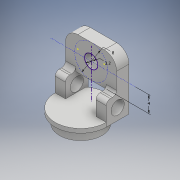
# Autodesk Inventor part: magnet-holder-end
Saved by Autodesk Inventor 2018 (Build 220112000, 112)
## iProperties
Created: 2025-03-13
Part Number: magnet-holder-end
Material: Generic
Document SubType Name: Modeling
Designer: neo
Density: 1 g/cm^3
Appearance: Default
Author: neo
Autodesk Inventor part; units mm, degrees
ref_plane "YZ Plane" through (0, 0, 0) normal (1, 0, 0) x (0, 1, 0)
ref_plane "XZ Plane" through (0, 0, 0) normal (0, 1, 0) x (-1, 0, 0)
ref_plane "XY Plane" through (0, 0, 0) normal (0, 0, 1) x (1, 0, 0)
sketch "Sketch1" plane through (0, 0, 0) normal (0, 0, 1) x (1, 0, 0)
  circle A0 centre (0, 0) radius 5.15
  dimension "d0" = 10.3
  constraints: 1 centre point, 1 coincident
  measures "d0" diameter of A0
extrude "Extrusion1" add sketch "Sketch1" along normal blind 2.3
sketch "Sketch2" plane through (0, 0, 2.3) normal (0, 0, 1) x (1, 0, 0)
  circle A0 centre (0, 0) radius 6.2
  dimension "d3" = 12.4
  constraints: 1 centre point, 1 coincident
  measures "d3" diameter of A0
extrude "Extrusion2" add sketch "Sketch2" along normal blind 1
sketch "Sketch3" plane through (0, 0, 2.3) normal (0, 0, -1) x (-1, 0, 0)
  circle A0 centre (0, 0) radius 6.2 construction
  line L0 (6.2, 0) -> (3.7, 0)
  line L1 (3.7, 0) -> (3.7, 5.5)
  line L2 (3.7, 5.5) -> (6.2, 5.5)
  line L3 (6.2, 5.5) -> (6.2, 0)
  line L4 (0, -6.2) -> (0, 6.2)
  circle A1 centre (0, 0) radius 6.2 construction
  line L5 (-6.2, 0) -> (-3.7, 0)
  line L6 (-3.7, 0) -> (-3.7, 5.5)
  line L7 (-3.7, 5.5) -> (-6.2, 5.5)
  line L8 (-6.2, 5.5) -> (-6.2, 0)
  dimension "d6" = 5.5
  dimension "d7" = 2.5
  constraints: 18 end point, 4 symmetric about line, 3 point on circle, 2 parallel, 1 horizontal, 1 horizontal alignment, 1 line through centre, 1 perpendicular, 1 vertical, 2 other
  measures "d6" distance of L2.end L0.start
  measures "d7" distance of L1.end L2.end
extrude "Extrusion3" add sketch "Sketch3" against normal blind 5.5
sketch "Sketch4" plane through (6.2, 0, 2.3) normal (1, 0, 0) x (0, 0, -1)
  line L0 (0, 5.5) -> (0, 0) construction
  line L1 (0, 5.5) -> (-5.5, 5.5) construction
  line L2 (-5.5, 0) -> (-5.5, 5.5) construction
  line L3 (-1, 0) -> (-5.5, 0) construction
  line L4 (0, 0) -> (-1, 0) construction
  line L5 (-5.5, 0) -> (-5.5, 5.5) construction
  line L6 (0, 5.5) -> (-5.5, 0) construction
  line L7 (0, -6.2) -> (0, 0) construction
  line L8 (-5.5, 5.5) -> (0, 0) construction
  circle A0 centre (-2.75, 2.75) radius 1.6
  point P0 (2.3, 0)
  dimension "d10" = 3.2
  constraints: 4 end point, 1 centre point, 1 midpoint
  measures "d10" diameter of A0
extrude "Extrusion4" cut sketch "Sketch4" against normal through all
fillet "Fillet1" radius 1 2 edges at (4.95, 0, 7.8) (-4.95, 0, 7.8)
sketch "Sketch5" plane through (0, 0, 7.8) normal (0, 0, 1) x (1, 0, 0)
  line L0 (6.2, 1) -> (3.7, 1) construction
  line L1 (6.2, 1) -> (6.2, 5.5) construction
  line L2 (6.2, 5.5) -> (3.7, 5.5) construction
  line L3 (3.7, 5.5) -> (3.7, 1) construction
  line L4 (-3.7, 1) -> (-6.2, 1) construction
  line L5 (-3.7, 1) -> (-3.7, 5.5) construction
  line L6 (-3.7, 5.5) -> (-6.2, 5.5) construction
  line L7 (-6.2, 5.5) -> (-6.2, 1) construction
  line L8 (6.2, 5.5) -> (6.2, 0) projected
  line L9 (-6.2, 5.5) -> (-6.2, 0) projected
  line L10 (6.2, 5.5) -> (-6.2, 5.5)
  line L11 (-6.2, 5.5) -> (-6.2, 2.5)
  line L12 (-6.2, 2.5) -> (6.2, 2.5)
  line L13 (6.2, 2.5) -> (6.2, 5.5)
  point P0 (0, 0)
  dimension "d14" = 3
  constraints: 8 end point, 2 parallel, 1 horizontal, 1 perpendicular, 1 point on line
  measures "d14" distance between parallel lines of L10 L12
extrude "Extrusion5" add sketch "Sketch5" along normal blind 8
fillet "Fillet2" radius 1 2 edges at (-4.95, 2.5, 7.8) (4.95, 2.5, 7.8)
fillet "Fillet3" radius 3 2 edges at (-6.2, 4, 15.8) (6.2, 4, 15.8)
sketch "Sketch6" plane through (-3.7, 2.5, 7.8) normal (0, -1, 0) x (1, 0, 0)
  line L0 (3.7, -7.8) -> (3.7, 7.2594)
  line L1 (0, 0) -> (7.4, 0) construction
  arc A0 (9.9, 5) -> (6.9, 8) centre (6.9, 5) ccw construction
  line L2 (0.5, 8) -> (6.9, 8) construction
  arc A1 (0.5, 8) -> (-2.5, 5) centre (0.5, 5) ccw construction
  line L3 (-2.5, 1) -> (-2.5, 5) construction
  line L4 (0, 1) -> (-2.5, 1) construction
  line L5 (0, 1) -> (0, 0) construction
  line L6 (0, 0) -> (7.4, 0) construction
  line L7 (7.4, 0) -> (7.4, 1) construction
  line L8 (9.9, 1) -> (7.4, 1) construction
  line L9 (9.9, 1) -> (9.9, 5) construction
  line L10 (-6.2522, 4) -> (14.3588, 4) construction
  circle A2 centre (3.7, 4) radius 1.6
  circle A3 centre (3.7, 4) radius 4 construction
  dimension "d19" = 4
  dimension "d20" = 3.2
  dimension "d23" = 8
  constraints: 4 end point, 2 centre point, 2 point on line, 1 coincident, 1 horizontal, 1 vertical
  measures "d19" distance between parallel lines of L1 L10
  measures "d20" diameter of A2
  measures "d23" diameter of A3
extrude "Extrusion6" cut sketch "Sketch6" against normal through all
body "Solid1"
